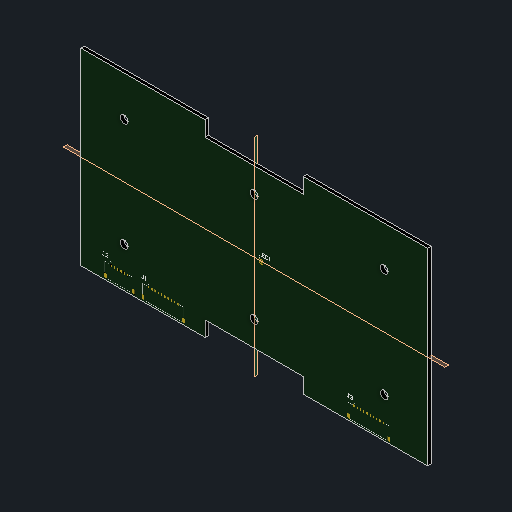
# Autodesk Inventor part: ledbrick_plus_led_BOARD
Saved by Autodesk Inventor 2026.1 (Build 301233020, 233B)
## iProperties
Created: 2025-09-21
Part Number: ledbrick_plus_led_BOARD
Material: Generic
Document SubType Name: Modeling
Designer: atrus
Density: 1 g/cm^3
Appearance: BoardColor
Author: atrus
Autodesk Inventor part; units mm, degrees
ref_plane "YZ Plane" through (0, 0, 0) normal (1, 0, 0) x (0, 1, 0)
ref_plane "XZ Plane" through (0, 0, 0) normal (0, 1, 0) x (-1, 0, 0)
ref_plane "XY Plane" through (0, 0, 0) normal (0, 0, 1) x (1, 0, 0)
ref_plane "BoardFrontPlane" through (0, 0, 0) normal (0, 0, 1) x (1, 0, 0)
sketch "Sketch1" plane through (0, 0, 0) normal (0, 0, 1) x (1, 0, 0)
  line L0 (26, 26) -> (186, 26)
  line L1 (186, 26) -> (186, 113)
  line L2 (186, 113) -> (26, 113)
  line L3 (26, 113) -> (26, 26)
  constraints: 8 end point
extrude "BoardOutline" add sketch "Sketch1" along normal blind 1.5957
ref_plane "Work Plane2" through (106, 26, 0) normal (-1, 0, 0) x (0, 0, 1)
ref_plane "Work Plane3" through (26, 69.5, 0) normal (0, 1, 0) x (1, 0, 0)
sketch "Sketch4" plane through (0, 0, 1.5957) normal (0, 0, 1) x (1, 0, 0)
  line L0 (83.3, 26) -> (83.3, 33.05)
  line L1 (83.3, 33.05) -> (128.7, 33.05)
  line L2 (128.7, 33.05) -> (128.7, 26)
  line L3 (26, 113) -> (26, 26) projected
  line L4 (83.3, 26) -> (128.7, 26)
  point P0 (83.3, 29.525)
  point P1 (186, 26)
  dimension "d9" = 57.3
  dimension "d10" = 57.3
  dimension "d11" = 7.05
  constraints: 8 end point, 1 horizontal, 1 midpoint
  measures "d9" distance from line of L3 point (83.3, 29.525)
  measures "d10" distance from line of point (186, 26) L2
  measures "d11" distance of L1.end L2.end
sketch "Sketch5" plane through (0, 0, 1.5957) normal (0, 0, 1) x (1, 0, 0)
  line L0 (128.7, 113) -> (128.7, 105.95)
  line L1 (128.7, 105.95) -> (83.3, 105.95)
  line L2 (83.3, 105.95) -> (83.3, 113)
  line L3 (83.3, 113) -> (128.7, 113)
  line L4 (186, 113) -> (26, 113) projected
  point P0 (83.3, 109.475)
  point P1 (128.7, 109.475)
  dimension "d12" = 57.3
  dimension "d13" = 57.3
  dimension "d14" = 7.05
  constraints: 8 end point, 2 midpoint, 1 collinear
  measures "d12" horizontal distance of point (83.3, 109.475) L4.end
  measures "d13" horizontal distance of L4.start point (128.7, 109.475)
  measures "d14" distance of L0.start L0.end
extrude "Extrusion3" cut sketch "Sketch5" against normal blind 10
extrude "Extrusion4" cut sketch "Sketch4" against normal blind 10
sketch "img_Top" plane through (0, 0, 1.5957) normal (0, 0, 1) x (1, 0, 0)
  line L0 (26, 113) -> (186, 113) construction
  line L1 (186, 113) -> (186, 26.0021) construction
  line L2 (186, 26.0021) -> (26, 26.0021) construction
  line L3 (26, 26.0021) -> (26, 113) construction
  constraints: 2 other
decal "Decal_Top"
sketch "Sketch8" plane through (0, 0, 1.5957) normal (0, 0, 1) x (1, 0, 0)
  point P0 (106, 94.5)
hole "Free-Hole1" at (106, 94.5, 1.5957) direction (0, 0, -1) diameter 3.6 end through all
sketch "Sketch9" plane through (0, 0, 1.5957) normal (0, 0, 1) x (1, 0, 0)
  point P0 (106, 44.5)
hole "Free-Hole1_2" at (106, 44.5, 1.5957) direction (0, 0, -1) diameter 3.6 end through all
sketch "Sketch11" plane through (0, 0, 1.5957) normal (0, 0, 1) x (1, 0, 0)
  point P0 (46, 94.5)
hole "Free-Hole4" at (46, 94.5, 1.5957) direction (0, 0, -1) diameter 3.6 end through all
sketch "Sketch12" plane through (0, 0, 1.5957) normal (0, 0, 1) x (1, 0, 0)
  point P0 (46, 44.5)
hole "Free-Hole4_2" at (46, 44.5, 1.5957) direction (0, 0, -1) diameter 3.6 end through all
sketch "Sketch13" plane through (0, 0, 1.5957) normal (0, 0, 1) x (1, 0, 0)
  point P0 (166, 44.5)
hole "Free-Hole4_3" at (166, 44.5, 1.5957) direction (0, 0, -1) diameter 3.6 end through all
sketch "Sketch14" plane through (0, 0, 1.5957) normal (0, 0, 1) x (1, 0, 0)
  point P0 (166, 94.5)
hole "Free-Hole4_4" at (166, 94.5, 1.5957) direction (0, 0, -1) diameter 3.6 end through all
body "Solid1"
